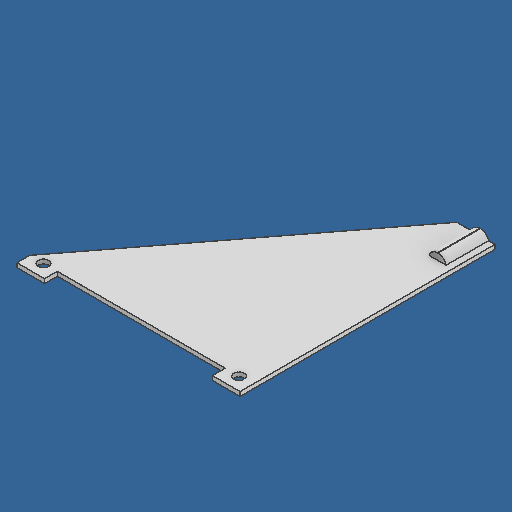
# Autodesk Inventor part: Triangle
Saved by Autodesk Inventor 2026.2 (Build 302298000, 298)
## iProperties
Created: 2025-12-09
Part Number: Triangle
Material: Generic
Document SubType Name: Modeling
Designer: Thoma
Density: 1 g/cm^3
Appearance: Default
Author: Thoma
Autodesk Inventor part; units mm, degrees
ref_plane "YZ Plane" through (0, 0, 0) normal (1, 0, 0) x (0, 1, 0)
ref_plane "XZ Plane" through (0, 0, 0) normal (0, 1, 0) x (-1, 0, 0)
ref_plane "XY Plane" through (0, 0, 0) normal (0, 0, 1) x (1, 0, 0)
sketch "Sketch1" plane through (0, 0, 0) normal (0, 1, 0) x (-1, 0, 0)
  line L0 (6.1765, 12) -> (-98.8235, 12)
  line L1 (-98.8235, 12) -> (-98.8235, -102)
  line L2 (-6.8235, 12) -> (-6.8235, 18)
  line L3 (-6.8235, 18) -> (6.1765, 18)
  line L4 (6.1765, 18) -> (6.1765, 12)
  line L5 (-98.8235, 12) -> (-98.8235, 18)
  line L6 (-98.8235, 18) -> (-85.8235, 18)
  line L7 (-85.8235, 18) -> (-85.8235, 12)
  line L8 (-98.8235, -102) -> (-85.8235, -87.8857)
  line L9 (-6.8235, -2.1143) -> (6.1765, 12)
  line L10 (-98.8235, -102) -> (-80.8235, -102)
  line L11 (6.1765, 12) -> (-80.8235, -102)
  point P0 (0, 0)
  point P1 (-96.8235, 18)
  point P2 (-96.8235, 18)
  dimension "d0" = 114
  dimension "d1" = 105
  dimension "d2" = 13
  dimension "d3" = 6
  dimension "d4" = 13
  dimension "d5" = 6
  dimension "d6" = 18
  constraints: 24 end point, 4 perpendicular, 4 point on line, 3 horizontal, 1 vertical
  measures "d0" distance of L0.end L1.end
  measures "d1" distance of L0.start L0.end
  measures "d2" distance of L2.start L0.start
  measures "d3" distance of L2.start L2.end
  measures "d4" distance of L5.end L6.end
  measures "d5" distance of L6.end L7.end
  measures "d6" distance of L1.end L10.end
extrude "Extrusion1" add sketch "Sketch1" along normal blind 2
sketch "Sketch2" plane through (0, 2, 0) normal (0, 1, 0) x (1, 0, 0)
  line L0 (98.8235, 102) -> (80.8235, 102) projected
  line L1 (95.8235, 102) -> (87.8235, 102)
  line L2 (87.8235, 102) -> (87.8235, 82)
  line L3 (87.8235, 82) -> (95.8235, 82)
  line L4 (95.8235, 82) -> (95.8235, 102)
  line L5 (98.8235, -18) -> (98.8235, 102) projected
  point P0 (0, 0)
  dimension "d9" = 20
  dimension "d10" = 8
  dimension "d11" = 3
  constraints: 8 end point, 2 parallel, 1 horizontal, 1 perpendicular, 1 point on line
  measures "d9" distance of L1.end L2.end
  measures "d10" distance of L2.end L3.end
  measures "d11" distance between parallel lines of L5 L4
extrude "Extrusion2" add sketch "Sketch2" along normal blind 3
fillet "Fillet1" radius 4 2 edges at (87.8235, 5, -92) (95.8235, 5, -92)
sketch "Sketch3" plane through (0, 0, 0) normal (0, -1, 0) x (1, 0, 0)
  line L0 (87.8235, -102) -> (80.8235, -102) projected
  line L1 (87.8235, -102) -> (95.8235, -102)
  line L2 (95.8235, -102) -> (95.8235, -82)
  line L3 (95.8235, -82) -> (87.8235, -82)
  line L4 (87.8235, -82) -> (87.8235, -102)
  line L5 (98.8235, 18) -> (98.8235, -102) projected
  point P0 (0, 0)
  dimension "d16" = 20
  dimension "d17" = 8
  dimension "d18" = 3
  constraints: 8 end point, 2 parallel, 1 horizontal, 1 perpendicular
  measures "d16" distance of L3.end L0.start
  measures "d17" distance of L2.end L3.end
  measures "d18" distance between parallel lines of L5 L2
extrude "Extrusion3" add sketch "Sketch3" along normal blind 3
fillet "Fillet3" radius 4 2 edges at (87.8235, -3, -92) (95.8235, -3, -92)
sketch "Sketch4" plane through (80.8235, 0, -102) normal (0, 0, -1) x (-1, 0, 0)
  arc A0 (-15, 0) -> (-11.127, -3) centre (-11.127, 1) ccw projected
  line L0 (-11.127, 4.8105) -> (-11.127, -3)
  circle A1 centre (-11.127, 1) radius 2.5
  point P0 (80.8235, 0)
  dimension "d25" = 5
  constraints: 2 end point, 1 centre point, 1 coincident, 1 vertical
  measures "d25" diameter of A1
extrude "Extrusion4" cut sketch "Sketch4" against normal blind 5
sketch "Sketch5" plane through (0, 2, 0) normal (0, 1, 0) x (1, 0, 0)
  line L0 (85.8235, -12) -> (85.8235, -18) projected
  line L1 (85.8235, -12) -> (98.8235, -12)
  line L2 (98.8235, -18) -> (98.8235, 102) projected
  circle A0 centre (92.3235, -12) radius 2.5
  point P0 (0, 0)
  dimension "d26" = 5
  constraints: 2 end point, 1 centre point, 1 horizontal, 1 midpoint, 1 point on line
  measures "d26" diameter of A0
extrude "Extrusion5" cut sketch "Sketch5" against normal blind 2
sketch "Sketch6" plane through (0, 2, 0) normal (0, 1, 0) x (1, 0, 0)
  line L0 (-6.1765, -12) -> (-6.1765, -18) projected
  line L1 (6.8235, -18) -> (6.8235, -12) projected
  line L2 (-6.1765, -12) -> (6.8235, -12)
  circle A0 centre (0.3235, -12) radius 2.5
  point P0 (0, 0)
  dimension "d29" = 5
  dimension "d32" = 6.5
  dimension "d33" = 6
  constraints: 2 end point, 1 centre point, 1 horizontal, 1 midpoint
  measures "d29" diameter of A0
  measures "d32" distance of L0.start A0.centre
  measures "d33" distance of L0.start L0.end
extrude "Extrusion6" cut sketch "Sketch6" against normal blind 2
equation "\"d23\" = d22"
equation "\"d22\" = 5"
body "Solid1"
